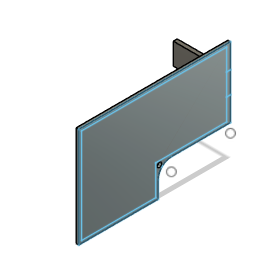
CaseAssembly v1 (Autodesk Fusion 360 archive; units mm, degrees)
design "Lid"
Autodesk Fusion 360 part; units mm, degrees
sketch "Sketch1" plane through (0, 0, 0) normal (1, 0, 0) x (0, 0, -1)
  line L0 (-50.8576, -27.0879) -> (-50.8576, 45.2121)
  line L1 (62.6424, 47.2121) -> (-52.8576, 47.2121)
  line L2 (59.6424, 28.8121) -> (62.6424, 28.8121)
  line L3 (62.6424, 28.8121) -> (62.6424, 47.2121)
  line L4 (59.6424, 12.3121) -> (59.6424, -4.0879)
  line L5 (59.6424, 45.2121) -> (59.6424, 28.8121)
  line L6 (-50.8576, 45.2121) -> (59.6424, 45.2121)
  line L7 (17.6424, -6.0879) -> (62.6424, -6.0879)
  line L8 (59.6424, -4.0879) -> (5.6424, -4.0879)
  line L9 (62.6424, 12.3121) -> (59.6424, 12.3121)
  line L10 (-52.8576, 47.2121) -> (-52.8576, -29.0879)
  line L11 (-52.8576, -29.0879) -> (7.6424, -29.0879)
  line L12 (5.6424, -27.0879) -> (-50.8576, -27.0879)
  line L13 (5.6424, -4.0879) -> (5.6424, -27.0879)
  line L14 (7.6424, -29.0879) -> (7.6424, -16.0879)
  line L15 (62.6424, -6.0879) -> (62.6424, 12.3121)
  line L16 (59.6424, 28.8121) -> (59.6424, 12.3121)
  line L17 (62.6424, 12.3121) -> (62.6424, 28.8121)
  arc A0 (17.6424, -6.0879) -> (7.6424, -16.0879) centre (17.6424, -16.0879) ccw
  point P0 (62.6424, -13.1879)
  dimension "d9" = 10
  constraint perpendicular L9 L16
  constraint perpendicular L2 L17
  constraint tangent L7 A0
  constraint tangent L14 A0
  measures "d9" radius of A0
extrude "Extrude1" add sketch "Sketch1" against normal blind 4 contours L0 L4 L5 L6 L8 L12 L13 L16
extrude "Extrude2" add sketch "Sketch1" against normal blind 2 contours L0 L1 L2 L3 L4 L5 L6 L7 L8 L9 L10 L11 L12 L13 L14 L15 A0
extrude "Extrude3" add sketch "Sketch1" against normal blind 40.55 contours L2 L9 L16 L17
sketch "Sketch3" plane through (0, 0, 0) normal (1, 0, 0) x (0, 0, -1)
  line L0 (62.6424, -6.0879) -> (62.6424, 47.2121)
  line L1 (62.6424, 47.2121) -> (-52.8576, 47.2121)
  line L2 (-52.8576, 47.2121) -> (-52.8576, -29.0879)
  line L3 (-52.8576, -29.0879) -> (7.6424, -29.0879)
  line L4 (7.6424, -29.0879) -> (7.6424, -16.0879)
  arc A0 (17.6424, -6.0879) -> (7.6424, -16.0879) centre (17.6424, -16.0879) ccw
  line L5 (17.6424, -6.0879) -> (62.6424, -6.0879)
  circle A1 centre (8.5297, -6.9752) radius 1.75
  line L6 (5.6424, -4.0879) -> (5.6424, -27.0879) construction
  line L7 (59.6424, -4.0879) -> (5.6424, -4.0879) construction
  line L8 (8.5297, -5.2252) -> (8.5297, -4.0879) construction
  line L9 (6.7797, -6.9752) -> (5.6424, -6.9752) construction
  line L10 (9.7672, -8.2126) -> (10.5714, -9.0168) construction
  point P0 (5.6424, -4.0879)
  dimension "d10" = 3.5
  constraint coincident A1 L8.start
  constraint coincident L7 L8.end
  constraint perpendicular L7 L8
  constraint coincident A1 L9.start
  constraint coincident L6 L9.end
  constraint perpendicular L6 L9
  constraint coincident A1 L10.start
  constraint midpoint A0 L10.end
  constraint vertical A1.centre L8.end
  constraint horizontal A1.centre L9.end
  constraint equal L8 L9
  constraint equal L9 L10
  constraint collinear A1.centre L10.start L10.end
  measures "d10" diameter of A1
extrude "Extrude4" cut sketch "Sketch3" against normal blind 2 contours A1
